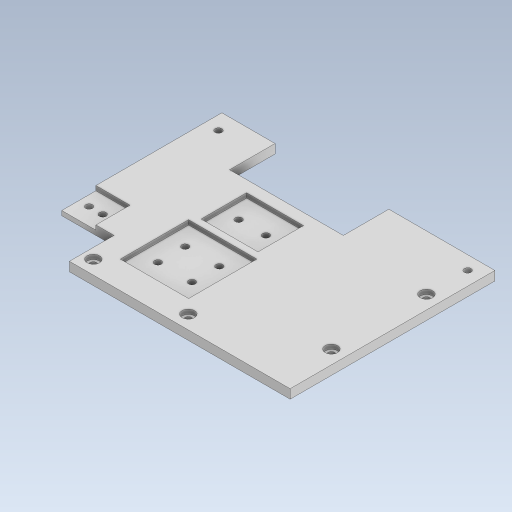
# Autodesk Inventor part: Casis Kanan Atas
Saved by Autodesk Inventor 2023.5 (Build 275446000, 446)
## iProperties
Created: 2025-09-16
Part Number: Casis Kanan Atas
Material: Generic
Document SubType Name: Modeling
Designer: Guntur
Density: 1 g/cm^3
Appearance: Default
Author: Guntur
## iProperties of the stored document Casis Kanan Atas_3DPrint.ipt
Created: 2025-09-19
Part Number: Casis Kanan Atas_3DPrint
Material: Generic
Document SubType Name: Modeling
Designer: Guntur
Density: 1 g/cm^3
Appearance: Default
Author: Guntur
Autodesk Inventor part; units mm, degrees
ref_plane "YZ Plane" through (0, 0, 0) normal (1, 0, 0) x (0, 1, 0)
ref_plane "XZ Plane" through (0, 0, 0) normal (0, 1, 0) x (-1, 0, 0)
ref_plane "XY Plane" through (0, 0, 0) normal (0, 0, 1) x (1, 0, 0)
sketch "Sketch1" plane through (0, 0, 0) normal (0, 1, 0) x (-1, 0, 0)
  line L0 (64.2199, -131.5556) -> (64.2199, -221.5556)
  line L1 (3.3449, -196.5556) -> (3.3449, -176.5556)
  circle A0 centre (9.8449, -186.5556) radius 1.5
  line L2 (-9.1551, -221.5556) -> (-9.1551, -201.5556)
  circle A1 centre (21.8449, -186.5556) radius 1.5
  line L3 (3.3449, -176.5556) -> (28.3449, -176.5556)
  line L4 (28.3449, -196.5556) -> (3.3449, -196.5556)
  line L5 (28.3449, -176.5556) -> (28.3449, -196.5556)
  line L6 (64.2199, -221.5556) -> (-55.7801, -221.5556)
  line L7 (-9.1551, -201.5556) -> (40.8449, -201.5556)
  line L8 (40.8449, -221.5556) -> (-9.1551, -221.5556)
  circle A2 centre (58.2199, -214.0556) radius 1.5
  line L9 (40.8449, -201.5556) -> (40.8449, -221.5556)
  line L10 (30.8449, -173.5556) -> (15.8449, -173.5556)
  line L11 (15.8449, -173.5556) -> (15.8449, -143.5556)
  line L12 (15.8449, -143.5556) -> (30.8449, -143.5556)
  line L13 (30.8449, -143.5556) -> (30.8449, -173.5556)
  line L14 (0.8449, -173.5556) -> (15.8449, -173.5556)
  circle A3 centre (8.3449, -164.5556) radius 1.5
  circle A4 centre (8.3449, -152.5556) radius 1.5
  circle A5 centre (23.3449, -164.5556) radius 1.5
  line L15 (0.8449, -143.5556) -> (0.8449, -173.5556)
  line L16 (15.8449, -173.5556) -> (15.8449, -143.5556)
  line L17 (15.8449, -143.5556) -> (0.8449, -143.5556)
  circle A6 centre (23.3449, -152.5556) radius 1.5
  line L18 (49.2199, -166.2056) -> (64.2199, -166.2056)
  circle A7 centre (53.7199, -158.7056) radius 1.5
  circle A8 centre (53.7199, -158.7056) radius 2.5
  circle A9 centre (59.7199, -158.7056) radius 1.5
  circle A10 centre (59.7199, -158.7056) radius 2.5
  line L19 (49.2199, -151.2056) -> (49.2199, -166.2056)
  line L20 (64.2199, -166.2056) -> (64.2199, -151.2056)
  line L21 (64.2199, -151.2056) -> (49.2199, -151.2056)
  line L22 (64.2199, -148.5556) -> (64.2199, -131.5556)
  line L23 (64.2199, -131.5556) -> (49.2199, -131.5556)
  line L24 (-55.7801, -221.5556) -> (-55.7801, -131.5556)
  line L25 (-55.7801, -131.5556) -> (-6.8176, -131.5556)
  line L26 (-55.7801, -176.5556) -> (-55.7801, -171.5556)
  line L27 (-55.7801, -171.5556) -> (-55.7801, -181.5556)
  circle A11 centre (-49.7801, -215.5556) radius 1.5
  circle A12 centre (-49.7801, -155.6806) radius 1.5
  circle A13 centre (-49.7801, -155.6806) radius 2.75
  line L28 (-41.5051, -176.5556) -> (-60.5551, -176.5556) construction
  circle A14 centre (-49.7801, -197.4306) radius 2.75
  circle A15 centre (-49.7801, -197.4306) radius 1.5
  line L29 (3.1824, -131.5556) -> (64.2199, -131.5556)
  circle A16 centre (36.7199, -137.5556) radius 2.75
  circle A17 centre (36.7199, -137.5556) radius 1.5
  line L30 (3.1824, -131.5556) -> (-6.8176, -131.5556)
  circle A18 centre (-5.0301, -137.5556) radius 1.5
  circle A19 centre (-5.0301, -137.5556) radius 2.75
  line L31 (15.8449, -176.5556) -> (15.8449, -139.0556) construction
  line L32 (49.2199, -151.2056) -> (41.2199, -151.2056)
  line L33 (41.2199, -151.2056) -> (41.2199, -131.5556)
  point P0 (0, -174.625)
  point P1 (-1.8176, -176.5556)
  point P2 (3.3449, -186.5556)
  point P3 (36.7199, -143.5556)
  point P4 (-5.0301, -143.5556)
  point P5 (-9.1551, -221.5556)
  point P6 (44.2199, -131.5556)
  dimension "d32" = 12
  dimension "d33" = 7.5
  dimension "d34" = 7.5
  dimension "d35" = 12
  dimension "d36" = 0
  dimension "d37" = 0
  dimension "d39" = 8
  dimension "d40" = 5.5
  dimension "d41" = 5.5
  dimension "d42" = 5.5
  dimension "d43" = 5.5
  constraints: 68 end point, 20 centre point, 6 coincident, 5 point on line, 2 vertical, 1 horizontal, 1 midpoint, 1 perpendicular
  measures "d32" distance of A6.centre A5.centre
  measures "d33" distance from line of L11 A5.centre
  measures "d34" distance from line of L16 A3.centre
  measures "d35" distance of A4.centre A3.centre
  measures "d36" distance between parallel lines of L31 L16
  measures "d37" distance between parallel lines of L16 L11
  measures "d39" distance of L19.start L32.end
  measures "d40" diameter of A14
  measures "d41" diameter of A13
  measures "d42" diameter of A19
  measures "d43" diameter of A16
extrude "Extrusion1" add sketch "Sketch1" along normal blind 4 contours L33 L32 L19 L18 L0 L6 L9 L7 L2 L24 L25 L30 L29
extrude "Extrusion2" add sketch "Sketch1" along normal blind 2 contours L0 L18 L19 L21 | L1 L3 L5 L4 | L10 L11 L12 L13 | L14 L15 L17 L11 | A8 | A10 | A13 | A14 | A16 | A19
body "Solid1"
